# Autodesk Inventor part: 0603YC104KATDA
Saved by Autodesk Inventor 2013 (Build 170138000, 138)
## iProperties
Created: 2013-01-27
Part Number: 0603YC104KATDA
Material: Generic
Document SubType Name: Modeling
Designer: davidgitz
Density: 1 g/cm^3
Author: davidgitz
Autodesk Inventor part; units mm, degrees
ref_plane "YZ Plane" through (0, 0, 0) normal (1, 0, 0) x (0, 1, 0)
ref_plane "XZ Plane" through (0, 0, 0) normal (0, 1, 0) x (-1, 0, 0)
ref_plane "XY Plane" through (0, 0, 0) normal (0, 0, 1) x (1, 0, 0)
sketch "SM0603, 0603YC104KATDA_48" plane through (0, 0, 0) normal (0, 0, 1) x (1, 0, 0)
  line L0 (-0.6731, 1.5621) -> (0.6731, 1.5621)
  line L1 (0.6731, 1.5621) -> (0.6731, -1.5621)
  line L2 (0.6731, -1.5621) -> (-0.6731, -1.5621)
  line L3 (-0.6731, -1.5621) -> (-0.6731, 1.5621)
  constraints: 8 end point
extrude "Extrusion1" add sketch "SM0603, 0603YC104KATDA_48" along normal blind 0.5999
body "Solid1"
